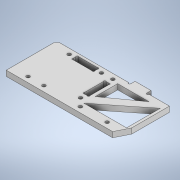
# Autodesk Inventor part: Trunk_lower_flank_frame_
Saved by Autodesk Inventor 2020.4 (Build 244396000, 396)
## iProperties
Created: 2022-01-02
Part Number: Trunk_lower_flank_frame_
Material: 一般
Document SubType Name: Modeling
Designer: Masato Kubotera
Density: 1 g/cm^3
Appearance: 既定
Author: Masato Kubotera
Autodesk Inventor part; units mm, degrees
ref_plane "YZ Plane" through (0, 0, 0) normal (1, 0, 0) x (0, 1, 0)
ref_plane "XZ Plane" through (0, 0, 0) normal (0, 1, 0) x (-1, 0, 0)
ref_plane "XY Plane" through (0, 0, 0) normal (0, 0, 1) x (1, 0, 0)
derived "Trunk_basis.ipt"
sketch "スケッチ1" plane through (0, 0, 0) normal (0, 1, 0) x (-1, 0, 0)
  line L0 (0, 24.5) -> (0, -139) construction
  circle A0 centre (5, 0) radius 10.5 construction
  line L1 (-7, 16) -> (36, 16) construction
  line L2 (36, 16) -> (36, -16) construction
  line L3 (36, -16) -> (-7, -16) construction
  line L4 (-7, -16) -> (-7, 16) construction
  line L5 (-7, 16) -> (36, -16) construction
  line L6 (36, 16) -> (-7, -16) construction
  line L7 (33, 13.5) -> (6, 13.5) construction
  line L8 (6, 13.5) -> (6, -13.5) construction
  line L9 (6, -13.5) -> (33, -13.5) construction
  line L10 (33, -13.5) -> (33, 13.5) construction
  line L11 (33, 13.5) -> (6, -13.5) construction
  line L12 (6, 13.5) -> (33, -13.5) construction
  line L13 (-7, 0) -> (36, 0) construction
  arc A1 (5, 16) -> (-7, 10.583) centre (5, 0) ccw construction
  line L14 (34.5651, -16.05) -> (5, -16.05)
  line L15 (5, 16.05) -> (34.5651, 16.05)
  line L16 (36.05, 14.5651) -> (36.05, -14.5651)
  line L17 (36.05, -16.05) -> (-7.05, 16.05) construction
  line L18 (-7.05, -16.05) -> (36.05, 16.05) construction
  arc A2 (5, 16.05) -> (-6.5314, 11.1638) centre (5, 0) ccw
  arc A3 (-6.5314, 11.1638) -> (-7.05, 9.8372) centre (-6.0721, 10.2196) ccw
  arc A4 (36.05, 14.5651) -> (34.5651, 16.05) centre (35.3075, 15.3075) ccw
  circle A5 centre (6, 13.5) radius 1.35 construction
  line L19 (19.5, 13.5) -> (19.5, -13.5) construction
  circle A6 centre (33, 13.5) radius 1.35 construction
  line L20 (-9.5, 24.5) -> (-14.5, 19.5)
  line L21 (-14.5, 19.5) -> (-14.5, 14.4295)
  line L22 (-14.5, 14.4295) -> (-28.5, -13.8021)
  line L23 (-28.5, -13.8021) -> (-28.5, -94.5)
  line L24 (86.5, -94.5) -> (86.5, -22)
  line L25 (86.5, -22) -> (52.05, -2.1103)
  line L26 (52.05, -2.1103) -> (52.05, 19.5)
  line L27 (52.05, 19.5) -> (47.05, 24.5)
  line L28 (47.05, 24.5) -> (-9.5, 24.5)
  line L29 (-22.6174, -92) -> (-28.5, -103.8625)
  line L30 (-28.5, -103.8625) -> (-28.5, -139)
  line L31 (-28.5, -139) -> (76.439, -139)
  line L32 (76.439, -139) -> (76.439, -92)
  line L33 (76.439, -92) -> (-22.6174, -92)
  line L34 (-16, -139) -> (-16, -99.5) construction
  line L35 (-16, -99.5) -> (16, -99.5) construction
  line L36 (16, -139) -> (16, -99.5) construction
  line L37 (-7.5, -139) -> (-7.5, -143)
  line L38 (-7.5, -143) -> (7.5, -143)
  line L39 (7.5, -139) -> (7.5, -143)
  arc A7 (-7.5, -139) -> (-9.6, -139) centre (-8.55, -139) ccw
  arc A8 (9.6, -139) -> (7.5, -139) centre (8.55, -139) ccw
  line L40 (-22.5, -139) -> (-22.5, -133) construction
  line L41 (-24, -133) -> (-21, -133) construction
  line L42 (-24, -133) -> (-24, -139) construction
  line L43 (-21, -133) -> (-21, -139) construction
  line L44 (-12, 22) -> (-7, 22) construction
  line L45 (-7, 22) -> (-7, -22) construction
  line L46 (-7, -22) -> (-12, -22) construction
  line L47 (-12, -22) -> (-12, 22) construction
  line L48 (-12, 22) -> (-7, -22) construction
  line L49 (-7, 22) -> (-12, -22) construction
  line L50 (-9.5, 22) -> (-9.5, -22) construction
  line L51 (-7, 0) -> (-12, 0) construction
  circle A9 centre (-9.5, 17.75) radius 1.6
  line L52 (-12, 10) -> (-9.5, 10) construction
  line L53 (-9.5, 10) -> (-9.5, -10) construction
  line L54 (-9.5, -10) -> (-12, -10) construction
  line L55 (-12, -10) -> (-12, 10) construction
  line L56 (-12, 10) -> (-9.5, -10) construction
  line L57 (-9.5, 10) -> (-12, -10) construction
  line L58 (-9.45, 10.05) -> (-12.05, 10.05)
  line L59 (-12.05, 7.95) -> (-12.05, -7.95)
  line L60 (-12.05, -10.05) -> (-9.45, -10.05)
  line L61 (-9.45, -7.95) -> (-9.45, 7.95)
  line L62 (-9.45, 10.05) -> (-12.05, -10.05) construction
  line L63 (-12.05, 10.05) -> (-9.45, -10.05) construction
  arc A10 (-12.05, 10.05) -> (-12.05, 7.95) centre (-12.05, 9) ccw
  line L64 (-10.75, 10) -> (-10.75, -10) construction
  arc A11 (-9.45, 7.95) -> (-9.45, 10.05) centre (-9.45, 9) ccw
  circle A12 centre (-9.5, -17.75) radius 1.6
  arc A13 (-12.05, -7.95) -> (-12.05, -10.05) centre (-12.05, -9) ccw
  arc A14 (-9.45, -10.05) -> (-9.45, -7.95) centre (-9.45, -9) ccw
  line L65 (36.05, 14.4) -> (44.55, 14.4) construction
  line L66 (44.55, 14.4) -> (44.55, -14.4) construction
  line L67 (36.05, -14.4) -> (44.55, -14.4) construction
  line L68 (47, 7.95) -> (47, -7.95)
  line L69 (49.55, 0) -> (44.55, 0) construction
  line L70 (44.55, 22) -> (49.55, 22) construction
  line L71 (49.6, -7.95) -> (49.6, 7.95)
  line L72 (48.3, 10) -> (48.3, -10) construction
  line L73 (49.55, 10) -> (47.05, -10) construction
  line L74 (49.55, -10) -> (47.05, -10) construction
  line L75 (49.55, 10) -> (49.55, -10) construction
  line L76 (47.05, 10) -> (49.55, -10) construction
  line L77 (47, -10.05) -> (49.6, -10.05)
  line L78 (47, 10.05) -> (49.6, -10.05) construction
  line L79 (49.6, 10.05) -> (47, -10.05) construction
  line L80 (49.55, -22) -> (44.55, -22) construction
  line L81 (44.55, 22) -> (49.55, -22) construction
  line L82 (49.55, 22) -> (49.55, -22) construction
  line L83 (49.55, 22) -> (44.55, -22) construction
  line L84 (47.05, 22) -> (47.05, -22) construction
  line L85 (44.55, -22) -> (44.55, 22) construction
  circle A15 centre (47.05, -17.75) radius 1.6
  arc A16 (49.6, -10.05) -> (49.6, -7.95) centre (49.6, -9) ccw
  line L86 (47.05, -10) -> (47.05, 10) construction
  arc A17 (47, -7.95) -> (47, -10.05) centre (47, -9) ccw
  arc A18 (47, 10.05) -> (47, 7.95) centre (47, 9) ccw
  arc A19 (49.6, 7.95) -> (49.6, 10.05) centre (49.6, 9) ccw
  line L87 (47.05, 10) -> (49.55, 10) construction
  line L88 (49.6, 10.05) -> (47, 10.05)
  circle A20 centre (47.05, 17.75) radius 1.6
  line L89 (-22.6174, -99.5) -> (-28.5, -94.5)
  line L90 (-22.6174, -99.5) -> (76.439, -99.5)
  circle A21 centre (61.1612, -97) radius 1.6
  line L91 (38.6653, -94.5) -> (68.939, -94.5) construction
  line L92 (68.939, -94.5) -> (68.939, -99.5) construction
  line L93 (68.939, -99.5) -> (38.6653, -99.5) construction
  line L94 (38.6653, -99.5) -> (38.6653, -94.5) construction
  line L95 (38.6653, -94.5) -> (68.939, -99.5) construction
  line L96 (68.939, -94.5) -> (38.6653, -99.5) construction
  line L97 (38.6653, -97) -> (68.939, -97) construction
  line L98 (-22.6174, -92) -> (-22.6174, -99.5) construction
  line L99 (53.8021, -99.5) -> (53.8021, -94.5) construction
  circle A22 centre (46.443, -97) radius 1.6
  line L100 (-28.5, -94.5) -> (86.5, -94.5) construction
  line L101 (86.5, -94.5) -> (76.439, -99.5)
  circle A23 centre (5, 0) radius 16 construction
  arc A24 (-6.5314, -11.1638) -> (5, -16.05) centre (5, 0) ccw
  arc A25 (-7.05, -9.8372) -> (-6.5314, -11.1638) centre (-6.0721, -10.2196) ccw
  arc A26 (34.5651, -16.05) -> (36.05, -14.5651) centre (35.3075, -15.3075) ccw
  line L102 (-7.05, -9.8372) -> (-7.05, 9.8372)
  line L103 (22.5, -139) -> (22.5, -133) construction
  line L104 (24, -133) -> (24, -139) construction
  line L105 (21, -133) -> (21, -139) construction
  line L106 (24, -133) -> (21, -133) construction
  circle A27 centre (6, -13.5) radius 1.35
  circle A28 centre (33, -13.5) radius 1.35
  line L107 (73.939, -139) -> (76.439, -136.5)
  line L108 (73.939, -94.5) -> (68.939, -94.5)
  line L109 (68.939, -94.5) -> (68.939, -139) construction
  line L110 (68.939, -139) -> (73.939, -139) construction
  line L111 (73.939, -139) -> (73.939, -94.5)
  line L112 (73.939, -94.5) -> (68.939, -139) construction
  line L113 (68.939, -94.5) -> (73.939, -139) construction
  line L114 (28.45, -104) -> (62.45, -104) construction
  line L115 (62.45, -104) -> (62.45, -127) construction
  line L116 (62.45, -127) -> (28.45, -127) construction
  line L117 (28.45, -127) -> (28.45, -104) construction
  line L118 (28.45, -104) -> (62.45, -127) construction
  line L119 (62.45, -104) -> (28.45, -127) construction
  line L120 (22, -131.5) -> (67.6513, -131.5) construction
  line L121 (67.6513, -131.5) -> (67.6513, -136.5) construction
  line L122 (67.6513, -136.5) -> (22, -136.5) construction
  line L123 (22, -136.5) -> (22, -131.5) construction
  line L124 (22, -131.5) -> (67.6513, -136.5) construction
  line L125 (67.6513, -131.5) -> (22, -136.5) construction
  line L126 (-26.0752, -133) -> (-26.0752, -101.4926)
  line L127 (-26.0752, -101.4926) -> (13.6883, -101.4926)
  line L128 (13.6883, -101.4926) -> (-26.0752, -133)
  line L129 (-15.4861, -133) -> (13.6883, -133)
  line L130 (13.6883, -133) -> (13.6883, -112.1048)
  line L131 (13.6883, -112.1048) -> (-15.4861, -133)
  line L132 (22, -99.5) -> (17, -99.5) construction
  line L133 (17, -99.5) -> (17, -139) construction
  line L134 (17, -139) -> (22, -139) construction
  line L135 (22, -139) -> (22, -99.5) construction
  line L136 (22, -99.5) -> (17, -139) construction
  line L137 (17, -99.5) -> (22, -139) construction
  line L138 (19.5, -99.5) -> (19.5, -139) construction
  circle A29 centre (19.5, -104.25) radius 1.6
  line L139 (17, -119.25) -> (22, -119.25) construction
  line L140 (-28.5, -139) -> (-28.5, -143) construction
  line L141 (-28.5, -143) -> (-7.5, -143) construction
  line L142 (28.5, -143) -> (7.5, -143) construction
  line L143 (28.5, -139) -> (28.5, -143) construction
  circle A30 centre (19.5, -134.25) radius 1.6
  line L144 (17, -109.25) -> (22, -109.25) construction
  line L145 (17, -129.25) -> (22, -129.25) construction
  line L146 (39.4409, -150.6176) -> (61.7571, -150.6176)
  line L147 (63.242, -152.1025) -> (63.242, -179.9354)
  line L148 (61.7571, -181.4204) -> (39.4409, -181.4204)
  line L149 (37.9559, -179.9354) -> (37.9559, -152.1025)
  line L150 (37.9559, -150.6176) -> (63.242, -181.4204) construction
  line L151 (63.242, -150.6176) -> (37.9559, -181.4204) construction
  arc A31 (39.4409, -150.6176) -> (37.9559, -152.1025) centre (38.6984, -151.36) ccw
  line L152 (50.599, -150.6176) -> (50.599, -181.4204) construction
  line L153 (37.9559, -166.019) -> (63.242, -166.019) construction
  arc A32 (63.242, -152.1025) -> (61.7571, -150.6176) centre (62.4995, -151.36) ccw
  arc A33 (37.9559, -179.9354) -> (39.4409, -181.4204) centre (38.6984, -180.6779) ccw
  arc A34 (61.7571, -181.4204) -> (63.242, -179.9354) centre (62.4995, -180.6779) ccw
  arc A35 (18.4349, -109.2) -> (16.95, -110.6849) centre (17.6925, -109.9425) ccw
  line L154 (18.4349, -109.2) -> (20.5651, -109.2)
  arc A36 (22.05, -110.6849) -> (20.5651, -109.2) centre (21.3075, -109.9425) ccw
  line L155 (16.95, -127.8151) -> (16.95, -110.6849)
  line L156 (16.95, -119.25) -> (22.05, -119.25) construction
  arc A37 (16.95, -127.8151) -> (18.4349, -129.3) centre (17.6925, -128.5575) ccw
  line L157 (19.5, -109.2) -> (19.5, -129.3) construction
  line L158 (16.95, -109.2) -> (22.05, -129.3) construction
  line L159 (22.05, -109.2) -> (16.95, -129.3) construction
  line L160 (20.5651, -129.3) -> (18.4349, -129.3)
  line L161 (22.05, -110.6849) -> (22.05, -127.8151)
  arc A38 (20.5651, -129.3) -> (22.05, -127.8151) centre (21.3075, -128.5575) ccw
  line L162 (44.8256, -131.5) -> (44.8256, -136.5) construction
  line L163 (34.8256, -131.5) -> (34.8256, -136.5) construction
  line L164 (67.6513, -134) -> (22, -134)
  circle A39 centre (29.8256, -134) radius 1.6
  arc A40 (54.8756, -132.9349) -> (53.3907, -131.45) centre (54.1332, -132.1925) ccw
  arc A41 (36.2606, -131.45) -> (34.7756, -132.9349) centre (35.5181, -132.1925) ccw
  line L165 (34.7756, -134) -> (54.8756, -134) construction
  line L166 (36.2606, -131.45) -> (53.3907, -131.45)
  line L167 (54.8756, -132.9349) -> (54.8756, -135.0651)
  line L168 (53.3907, -136.55) -> (36.2606, -136.55)
  line L169 (34.7756, -135.0651) -> (34.7756, -132.9349)
  line L170 (34.7756, -131.45) -> (54.8756, -136.55) construction
  line L171 (54.8756, -131.45) -> (34.7756, -136.55) construction
  line L172 (44.8256, -131.45) -> (44.8256, -136.55) construction
  arc A42 (34.7756, -135.0651) -> (36.2606, -136.55) centre (35.5181, -135.8075) ccw
  arc A43 (53.3907, -136.55) -> (54.8756, -135.0651) centre (54.1332, -135.8075) ccw
  line L173 (54.8256, -131.5) -> (54.8256, -136.5) construction
  circle A44 centre (59.8256, -134) radius 1.6
  circle A45 centre (-12.5, -97) radius 1.6
  circle A46 centre (12.5, -97) radius 1.6
  point P0 (0, 0)
  point P1 (14.5, 0)
  point P2 (19.5, 0)
  point P3 (-7.05, 10.6019)
  point P4 (19.5, 0)
  point P5 (-9.5, 0)
  point P6 (-10.75, 0)
  point P7 (48.3, 0)
  point P8 (47.05, 0)
  point P9 (53.8021, -97)
  point P10 (71.439, -116.75)
  point P11 (45.45, -115.5)
  point P12 (44.8256, -134)
  point P13 (19.5, -119.25)
  point P14 (50.599, -166.019)
  point P15 (19.5, -119.25)
  point P16 (19.5, -119.25)
  point P17 (44.8256, -134)
  point P18 (44.8256, -134)
  dimension "d4" = 45
  measures "d4" distance of L103.start L40.start
extrude "押し出し1" add sketch "スケッチ1" along normal blind 5 contours L89 L90 L111 L31 A8 A7 L30 L29 | L29 L33 L32 L90 L89 | L32 L107 L111 L90 | L31 L39 L38 L37
sketch "スケッチ2" plane through (28.5, 0, -139) normal (0, 0, -1) x (-1, 0, 0)
  line L0 (0, 0) -> (0, 5) projected
  line L1 (0, 2.5) -> (104.939, 2.5)
  line L2 (28.5, 0) -> (28.5, 5)
  line L3 (21, 5) -> (36, 5) projected
  point P0 (6, 2.5)
  point P1 (51, 2.5)
  dimension "d3" = 45
  constraints: 4 end point, 2 midpoint, 1 point on line, 1 symmetric about line, 1 vertical
  measures "d3" distance of point (51, 2.5) point (6, 2.5)
hole "穴1" at (22.5, 2.5, -139) at (-22.5, 2.5, -139) direction (0, 0, 1) diameter 2.459 depth 6 tip angle 118 thread size "M3x0.5" class "6H" standard "ISO Metric profile"
equation "\"d3\" = d4"
